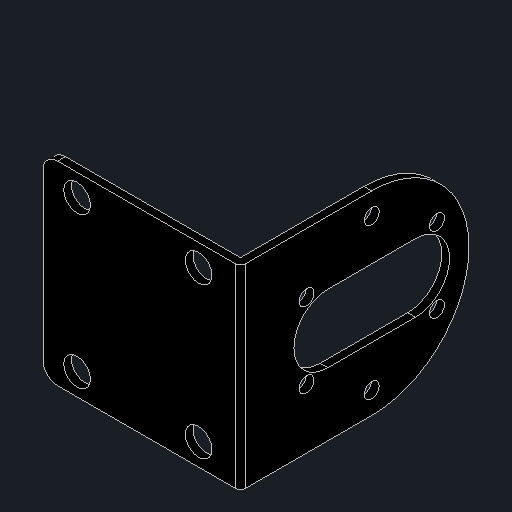
# Autodesk Inventor part: motor_connector
Saved by Autodesk Inventor 2026.1 (Build 301233020, 233B)
## iProperties
Created: 2025-11-17
Part Number: motor_connector
Material: 알루미늄 6061
Document SubType Name: Modeling
Designer: jaewook
Density: 2.7 g/cm^3
Appearance: 알루미늄 - 평지
Author: jaewook
Autodesk Inventor part; units mm, degrees
ref_plane "YZ Plane" through (0, 0, 0) normal (1, 0, 0) x (0, 1, 0)
ref_plane "XZ Plane" through (0, 0, 0) normal (0, 1, 0) x (-1, 0, 0)
ref_plane "작업 평면1" through (0, 0, 0) normal (0, 0, 1) x (1, 0, 0)
sketch "스케치1" plane through (0, 0, 0) normal (0, 0, 1) x (1, 0, 0)
  line L0 (130, -172.5) -> (91, -172.5)
  line L1 (91, -172.5) -> (91, -132.5)
  line L2 (91, -132.5) -> (130, -132.5)
  line L3 (130, -132.5) -> (130, -172.5)
  line L4 (91, -152.5) -> (130, -152.5) construction
  circle A0 centre (98, -168) radius 2.75
  line L5 (110.5, -172.5) -> (110.5, -132.5) construction
  circle A1 centre (98, -137) radius 2.75
  circle A2 centre (123, -168) radius 2.75
  circle A3 centre (123, -137) radius 2.75
  circle A4 centre (0, 170) radius 2 projected
  circle A5 centre (-73.6122, 42.5) radius 2 projected
  circle A6 centre (73.6122, 42.5) radius 2 projected
  line L6 (-175, 220) -> (-175, 200) projected
  line L7 (-175, 200) -> (-130, 200) projected
  line L8 (-130, 200) -> (-130, 105) projected
  line L9 (-130, 105) -> (-175, 105) projected
  line L10 (-175, 105) -> (-175, -105) projected
  line L11 (-175, -105) -> (-130, -105) projected
  line L12 (-130, -105) -> (-130, -200) projected
  line L13 (-130, -200) -> (-175, -200) projected
  line L14 (-175, -200) -> (-175, -220) projected
  arc A7 (-175, -220) -> (-145, -250) centre (-145, -220) ccw projected
  line L15 (-145, -250) -> (145, -250) projected
  arc A8 (145, -250) -> (175, -220) centre (145, -220) ccw projected
  line L16 (175, -220) -> (175, -200) projected
  line L17 (175, -200) -> (130, -200) projected
  line L18 (130, -200) -> (130, -105) projected
  line L19 (130, -105) -> (175, -105) projected
  line L20 (175, -105) -> (175, 105) projected
  line L21 (175, 105) -> (130, 105) projected
  line L22 (130, 105) -> (130, 200) projected
  line L23 (130, 200) -> (175, 200) projected
  line L24 (175, 200) -> (175, 220) projected
  arc A9 (175, 220) -> (145, 250) centre (145, 220) ccw projected
  line L25 (145, 250) -> (-145, 250) projected
  arc A10 (-145, 250) -> (-175, 220) centre (-145, 220) ccw projected
  circle A11 centre (-123, 166.7672) radius 2 projected
  circle A12 centre (122.9975, 135.7594) radius 2 projected
  circle A13 centre (97.9975, -135.761) radius 2 projected
  circle A14 centre (15.5, 71.3) radius 2 projected
  circle A15 centre (165.0067, -210) radius 2.5 projected
  circle A16 centre (119.0003, -180.2596) radius 1.25 projected
  circle A17 centre (-119, -122.2672) radius 1.25 projected
  circle A18 centre (-123, -135.7672) radius 2 projected
  circle A19 centre (0.0196, 140) radius 2 projected
  circle A20 centre (-123, -166.7672) radius 2 projected
  circle A21 centre (-70, -122.2672) radius 1.25 projected
  circle A22 centre (69.9966, -122.2627) radius 1.25 projected
  circle A23 centre (-165, 0) radius 2.5 projected
  circle A24 centre (-165.0067, 210) radius 2.5 projected
  circle A25 centre (-15.5, 119.1) radius 2 projected
  circle A26 centre (97.9995, -166.761) radius 2 projected
  circle A27 centre (97.9995, 166.761) radius 2 projected
  circle A28 centre (-98, 166.7672) radius 2 projected
  circle A29 centre (-123, 135.7672) radius 2 projected
  circle A30 centre (97.9975, 135.761) radius 2 projected
  circle A31 centre (122.9975, -135.7594) radius 2 projected
  circle A32 centre (-15.5, 71.3) radius 2 projected
  circle A33 centre (-164.9933, -210) radius 2.5 projected
  circle A34 centre (70.0003, -180.2627) radius 1.25 projected
  circle A35 centre (-119, -180.2672) radius 1.25 projected
  circle A36 centre (-98, -135.7672) radius 2 projected
  circle A37 centre (47.6216, 57.483) radius 2 projected
  circle A38 centre (-47.6412, 57.517) radius 2 projected
  circle A39 centre (-98, -166.7672) radius 2 projected
  circle A40 centre (-70, -180.2672) radius 1.25 projected
  circle A41 centre (118.9966, -122.2596) radius 1.25 projected
  circle A42 centre (165, 0) radius 2.5 projected
  circle A43 centre (164.9933, 210) radius 2.5 projected
  circle A44 centre (15.5, 119.1) radius 2 projected
  circle A45 centre (122.9995, -166.7594) radius 2 projected
  circle A46 centre (122.9995, 166.7594) radius 2 projected
  circle A47 centre (-98, 135.7672) radius 2 projected
  line L26 (-110, 97.5) -> (-93, 97.5) projected
  line L27 (-93, 97.5) -> (-93, 89.5) projected
  line L28 (-93, 89.5) -> (-110, 89.5) projected
  line L29 (-110, 89.5) -> (-110, 97.5) projected
  circle A48 centre (148, -23.75) radius 2 projected
  circle A49 centre (130.626, -27.584) radius 1.5 projected
  circle A50 centre (118.5, 61.5) radius 1.5 projected
  circle A51 centre (-118.5, 61.5) radius 1.5 projected
  circle A52 centre (21, -158.9548) radius 2 projected
  circle A53 centre (-22, -53) radius 2 projected
  circle A54 centre (-49.5, -194.9548) radius 2 projected
  circle A55 centre (-49.5, -158.9548) radius 2 projected
  circle A56 centre (21, -194.9548) radius 2 projected
  circle A57 centre (-155, 25) radius 1.5 projected
  circle A58 centre (118.5, 25) radius 1.5 projected
  circle A59 centre (123.133, -76) radius 1.5 projected
  circle A60 centre (37, -84) radius 2 projected
  line L30 (-93, -89.5) -> (-93, -97.5) projected
  line L31 (-93, -97.5) -> (-110, -97.5) projected
  line L32 (-110, -97.5) -> (-110, -89.5) projected
  line L33 (-110, -89.5) -> (-93, -89.5) projected
  circle A61 centre (-130, 5) radius 6 projected
  line L34 (110, 89.5) -> (93, 89.5) projected
  line L35 (93, 89.5) -> (93, 97.5) projected
  line L36 (93, 97.5) -> (110, 97.5) projected
  line L37 (110, 97.5) -> (110, 89.5) projected
  circle A62 centre (148, -84) radius 2 projected
  circle A63 centre (47.999, -27.584) radius 1.5 projected
  circle A64 centre (155, 61.5) radius 1.5 projected
  circle A65 centre (-155, 61.5) radius 1.5 projected
  circle A66 centre (49.5, -158.9548) radius 2 projected
  circle A67 centre (-86, -93.5) radius 2 projected
  circle A68 centre (-21, -194.9548) radius 2 projected
  circle A69 centre (-150, -53) radius 2 projected
  circle A70 centre (-21, -158.9548) radius 2 projected
  circle A71 centre (49.5, -194.9548) radius 2 projected
  circle A72 centre (-118.5, 25) radius 1.5 projected
  circle A73 centre (155, 25) radius 1.5 projected
  circle A74 centre (48, -76) radius 1.5 projected
  circle A75 centre (37, -23.75) radius 2 projected
  line L38 (110, -89.5) -> (110, -97.5) projected
  line L39 (110, -97.5) -> (93, -97.5) projected
  line L40 (93, -97.5) -> (93, -89.5) projected
  line L41 (93, -89.5) -> (110, -89.5) projected
  circle A76 centre (-70, 5) radius 6 projected
  circle A77 centre (0, -216.4634) radius 1.5 projected
  circle A78 centre (28.4775, -136.4634) radius 1.5 projected
  circle A79 centre (-28.4775, -136.4634) radius 1.5 projected
  point P0 (0, 0)
  dimension "d0" = 40
  dimension "d1" = 39
  dimension "d5" = 5.5
  dimension "d6" = 7
  dimension "d7" = 4.5
  dimension "d22" = 97.5
  constraints: 12 end point, 4 centre point, 4 midpoint, 3 symmetric about line, 2 parallel, 1 collinear, 1 horizontal, 1 perpendicular, 3 other
  measures "d0" distance of L0.end L1.end
  measures "d1" distance of L1.end L2.end
  measures "d5" diameter of A0
  measures "d6" distance from line of A0.centre L1
  measures "d7" distance from line of L0 A0.centre
  measures "d22" distance between parallel lines of L15 L4
extrude "돌출1" add sketch "스케치1" along normal blind 1.6 contours L0 L1 L2 L3 | A0 A26 | A1 A13 | A2 A45 | A3 A31 picked at (98.3703, -165.1311) picked at (98.3657, -134.1305) picked at (122.627, -165.1309) picked at (123.3661, -134.13)
sketch "스케치2" plane through (130, -172.5, 0) normal (1, 0, 0) x (0, 0, -1)
  line L0 (0, 40) -> (-1.6, 40)
  line L1 (-1.6, 0) -> (25.4, 0)
  line L2 (45.4, 20) -> (45.4, 20)
  line L3 (25.4, 40) -> (-1.6, 40)
  line L4 (-1.6, 40) -> (-1.6, 0)
  arc A0 (25.4, 0) -> (45.4, 20) centre (25.4, 20) ccw
  arc A1 (45.4, 20) -> (25.4, 40) centre (25.4, 20) ccw
  circle A2 centre (25.4, 35.5) radius 1.55
  circle A3 centre (11.9766, 27.75) radius 1.55
  circle A4 centre (11.9766, 12.25) radius 1.55
  circle A5 centre (25.4, 4.5) radius 1.55
  circle A6 centre (38.8234, 12.25) radius 1.55
  circle A7 centre (38.8234, 27.75) radius 1.55
  line L5 (34.4, 20) -> (16.4, 20) construction
  line L6 (34.4, 27) -> (16.4, 27)
  line L7 (16.4, 13) -> (34.4, 13)
  arc A8 (34.4, 13) -> (34.4, 27) centre (34.4, 20) ccw
  arc A9 (16.4, 27) -> (16.4, 13) centre (16.4, 20) ccw
  line L8 (0, 40) -> (-1.6, 40) projected
  point P0 (0, 172.5)
  point P1 (45.4, 40)
  point P2 (45.4, 20)
  point P3 (-1.6, 40)
  point P4 (0, 40)
  dimension "d3" = 1.6
  dimension "d8" = 47
  dimension "d9" = 20
  dimension "d10" = 3.1
  dimension "d11" = 15.5
  dimension "d14" = 360
  dimension "d16" = 9
  dimension "d17" = 14
  constraints: 18 end point, 10 centre point, 8 point on circle, 8 tangent, 3 parallel, 2 horizontal, 2 point on line, 1 collinear, 1 concentric, 1 midpoint, 1 perpendicular, 1 vertical alignment, 13 other
  measures "d8" distance of L3.end point (45.4, 40)
  measures "d9" radius of A0
  measures "d10" diameter of A2
  measures "d11" distance of A0.centre A2.centre
  measures "d16" distance of A1.centre L5.end
  measures "d17" diameter of A9
extrude "돌출2" add sketch "스케치2" along normal blind 1.6
fillet "모깎기1" radius 3 2 edges at (91, -132.5, 0.8) (91, -172.5, 0.8)
fillet "모깎기2" radius 1 1 edges at (131.6, -152.5, 1.6)
